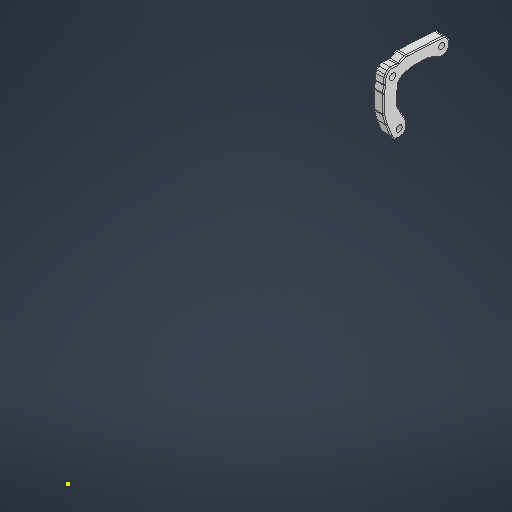
# Autodesk Inventor part: Lankarm_1
Saved by Autodesk Inventor 2026 (Build 300175000, 175)
## iProperties
Created: 2025-04-29
Part Number: Lankarm_1
Material: Generic
Document SubType Name: Modeling
Designer: elias
Density: 1 g/cm^3
Appearance: Default
Author: elias
Autodesk Inventor part; units mm, degrees
ref_plane "YZ Plane" through (0, 0, 0) normal (1, 0, 0) x (0, 1, 0)
ref_plane "XZ Plane" through (0, 0, 0) normal (0, 1, 0) x (-1, 0, 0)
ref_plane "XY Plane" through (0, 0, 0) normal (0, 0, 1) x (1, 0, 0)
sketch "Sketch1" plane through (0, 0, 0) normal (1, 0, 0) x (0, 1, 0)
  line L0 (3056.2025, 0) -> (3056.2025, -6694.5386) construction
  line L1 (3056.2025, -6694.5386) -> (0, -6694.5386) construction
  line L2 (0, -6694.5386) -> (0, 0) construction
  line L3 (0, 0) -> (3056.2025, 0) construction
  point P0 (0, 0)
  constraints: 2 end point, 2 other
sketch "Sketch2" plane through (0, 0, 0) normal (1, 0, 0) x (0, 1, 0)
  point P0 (0, 0)
sketch "Sketch3" plane through (0, 0, 0) normal (1, 0, 0) x (0, 1, 0)
  line L0 (939.4555, -1794.3559) -> (929.0384, -1814.0934)
  line L1 (929.0384, -1814.0934) -> (929.0384, -1838.2171)
  line L2 (929.0384, -1838.2171) -> (948.9738, -1861.2515)
  line L3 (948.9738, -1861.2515) -> (986.8041, -1861.2515)
  line L4 (986.8041, -1861.2515) -> (1011.9885, -1839.4555)
  line L5 (1011.9885, -1839.4555) -> (1020.3676, -1686.9006)
  line L6 (1020.3676, -1686.9006) -> (1022.4821, -1648.404)
  line L7 (1022.4821, -1648.404) -> (1006.0575, -1607.6637)
  line L8 (1006.0575, -1607.6637) -> (1008.4657, -1563.8186)
  line L9 (1008.4657, -1563.8186) -> (984.0611, -1543.1548)
  line L10 (984.0611, -1543.1548) -> (947.5988, -1541.1521)
  line L11 (947.2937, -1629.7597) -> (957.7072, -1685.4897)
  line L12 (957.7072, -1685.4897) -> (956.0216, -1746.9264)
  line L13 (956.0216, -1746.9264) -> (947.2937, -1779.5044)
  line L14 (947.2937, -1779.5044) -> (939.4555, -1794.3559)
  circle A0 centre (966.552, -1580.7994) radius 15
  circle A1 centre (975.9873, -1822.3056) radius 15
  line L15 (947.5988, -1541.1521) -> (915.0451, -1534.407)
  line L16 (915.0451, -1534.407) -> (824.7933, -1534.407)
  line L17 (824.7933, -1534.407) -> (773.8544, -1550.013)
  line L18 (773.8544, -1550.013) -> (714.4603, -1572.1504)
  line L19 (714.4603, -1572.1504) -> (692.203, -1588.4552)
  line L20 (692.203, -1588.4552) -> (685.7186, -1612.659)
  line L21 (685.7186, -1612.659) -> (693.6262, -1638.4699)
  line L22 (693.6262, -1638.4699) -> (709.0076, -1650.7852)
  line L23 (709.0076, -1650.7852) -> (743.987, -1650.7852)
  line L24 (743.987, -1650.7852) -> (771.9965, -1635.7735)
  line L25 (771.9965, -1635.7735) -> (830.34, -1604.5044)
  line L26 (830.34, -1604.5044) -> (872.2606, -1604.5044)
  line L27 (872.2606, -1604.5044) -> (924.5185, -1609.871)
  line L28 (924.5185, -1609.871) -> (947.2937, -1629.7597)
  circle A2 centre (728.4634, -1612.659) radius 15
  point P0 (0, 0)
  dimension "d14" = 30
  dimension "d15" = 30
  dimension "d20" = 30
  constraints: 58 end point, 4 perpendicular, 3 centre point, 3 parallel, 3 point on line, 1 collinear, 1 horizontal, 1 vertical
  measures "d14" diameter of A0
  measures "d15" diameter of A1
  measures "d20" diameter of A2
extrude "Extrusion2" add sketch "Sketch3" along normal mid plane 50
fillet "Fillet1" radius 20 26 edges at (0, 1008.4657, -1563.8186) (0, 1006.0575, -1607.6637) (0, 1022.4821, -1648.404) (0, 984.0611, -1543.1548) (0, 947.5988, -1541.1521) (0, 915.0451, -1534.407) (0, 824.7933, -1534.407) (0, 1011.9885, -1839.4555) (0, 986.8041, -1861.2515) (0, 948.9738, -1861.2515) (0, 929.0384, -1838.2171) (0, 929.0384, -1814.0934) (0, 947.2937, -1779.5044) (0, 956.0216, -1746.9264) (0, 957.7072, -1685.4897) (0, 947.2937, -1629.7597) (0, 773.8544, -1550.013) (0, 714.4603, -1572.1504) (0, 692.203, -1588.4552) (0, 685.7186, -1612.659) (0, 693.6262, -1638.4699) (0, 709.0076, -1650.7852) (0, 743.987, -1650.7852) (0, 830.34, -1604.5044) (0, 872.2606, -1604.5044) (0, 924.5185, -1609.871)
fillet "Fillet2" radius 5 96 edges at (-25, 1017.3459, -1741.9161) (25, 1017.3459, -1741.9161) (-25, 1010.4392, -1838.6953) (-25, 999.0058, -1850.6915) (-25, 986.335, -1859.9926) (-25, 968.733, -1861.2515) (-25, 949.801, -1859.4417) (-25, 938.4538, -1849.0961) (-25, 930.2973, -1837.7479) (-25, 929.0384, -1824.9058) (-25, 929.6251, -1814.2387) (-25, 938.7976, -1795.6024) (-25, 947.1765, -1779.4585) (-25, 951.6439, -1763.2666) (-25, 955.885, -1746.9065) (-25, 956.8675, -1716.0958) (-25, 957.5945, -1685.4986) (-25, 952.9425, -1659.9902) (-25, 935.6855, -1619.6228) (-25, 895.7371, -1606.9153) (-25, 872.2593, -1604.5305) (-25, 853.299, -1604.5044) (-25, 787.1635, -1627.6448) (-25, 743.8358, -1650.1831) (-25, 727.4965, -1650.7852) (-25, 709.4038, -1649.6564) (-25, 700.9846, -1644.3615) (-25, 694.3954, -1637.9476) (-25, 689.6097, -1625.3598) (-25, 686.5261, -1612.6447) (-25, 688.7929, -1601.1839) (-25, 693.1953, -1589.1343) (-25, 705.0525, -1579.0422) (-25, 714.551, -1572.3188) (-25, 745.4562, -1560.5976) (-25, 824.8263, -1534.6275) (-25, 797.892, -1542.6486) (-25, 870.3916, -1534.407) (-25, 915.0344, -1534.5112) (-25, 931.5927, -1537.8356) (-25, 947.606, -1541.0966) (-25, 963.2257, -1542.0104) (-25, 983.6556, -1544.1738) (-25, 995.0294, -1552.4419) (-25, 1006.3192, -1564.7431) (-25, 1007.1109, -1588.4846) (-25, 1006.5405, -1607.5837) (-25, 1014.2698, -1628.0339) (-25, 1021.9991, -1648.484) (25, 1021.9991, -1648.484) (25, 1014.2698, -1628.0339) (25, 1006.5405, -1607.5837) (25, 1007.1109, -1588.4846) (25, 1006.3192, -1564.7431) (25, 995.0294, -1552.4419) (25, 983.6556, -1544.1738) (25, 963.2257, -1542.0104) (25, 947.606, -1541.0966) (25, 931.5927, -1537.8356) (25, 915.0344, -1534.5112) (25, 870.3916, -1534.407) (25, 824.8263, -1534.6275) (25, 797.892, -1542.6486) (25, 714.551, -1572.3188) (25, 745.4562, -1560.5976) (25, 705.0525, -1579.0422) (25, 693.1953, -1589.1343) (25, 688.7929, -1601.1839) (25, 686.5261, -1612.6447) (25, 689.6097, -1625.3598) (25, 694.3954, -1637.9476) (25, 700.9846, -1644.3615) (25, 709.4038, -1649.6564) (25, 727.4965, -1650.7852) (25, 743.8358, -1650.1831) (25, 787.1635, -1627.6448) (25, 853.299, -1604.5044) (25, 872.2593, -1604.5305) (25, 895.7371, -1606.9153) (25, 935.6855, -1619.6228) (25, 952.9425, -1659.9902) (25, 957.5945, -1685.4986) (25, 956.8675, -1716.0958) (25, 955.885, -1746.9065) (25, 951.6439, -1763.2666) (25, 947.1765, -1779.4585) (25, 938.7976, -1795.6024) (25, 929.6251, -1814.2387) (25, 929.0384, -1824.9058) (25, 930.2973, -1837.7479) (25, 938.4538, -1849.0961) (25, 949.801, -1859.4417) (25, 968.733, -1861.2515) (25, 986.335, -1859.9926) (25, 999.0058, -1850.6915) (25, 1010.4392, -1838.6953)
body "Solid2"
